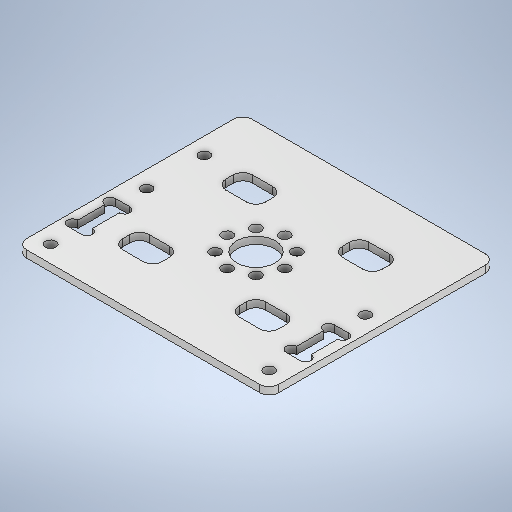
# Autodesk Inventor part: kosi_v3_1.5
Saved by Autodesk Inventor 2025.1 (Build 291241000, 241)
## iProperties
Created: 2024-09-01
Part Number: kosi_v3_1.5
Material: アルミニウム 2014-T4
Document SubType Name: Modeling
Designer: right
Density: 2.8 g/cm^3
Appearance: サテン
Mass: 8.90993 g
Surface Area: 49.4612 cm^2
Volume: 3.18212 cm^3
Author: right
Autodesk Inventor part; units mm, degrees
ref_plane "YZ Plane" through (0, 0, 0) normal (1, 0, 0) x (0, 1, 0)
ref_plane "XZ Plane" through (0, 0, 0) normal (0, 1, 0) x (-1, 0, 0)
ref_plane "XY Plane" through (0, 0, 0) normal (0, 0, 1) x (1, 0, 0)
sketch "スケッチ1" plane through (0, 0, 0) normal (0, 1, 0) x (-1, 0, 0)
  circle A0 centre (0, 0) radius 4
  circle A1 centre (0, 0) radius 8
  circle A2 centre (0, 0) radius 6 construction
  circle A3 centre (0, -6) radius 1.1
  circle A4 centre (4.2426, -4.2426) radius 1.1
  circle A5 centre (6, 0) radius 1.1
  circle A6 centre (4.2426, 4.2426) radius 1.1
  circle A7 centre (0, 6) radius 1.1
  circle A8 centre (-4.2426, 4.2426) radius 1.1
  circle A9 centre (-6, 0) radius 1.1
  circle A10 centre (-4.2426, -4.2426) radius 1.1
  line L0 (26.25, -23.5) -> (-26.25, -23.5)
  line L1 (-26.25, -23.5) -> (-26.25, 23.5)
  line L2 (-26.25, 23.5) -> (26.25, 23.5)
  line L3 (26.25, 23.5) -> (26.25, -23.5)
  line L4 (26.25, -23.5) -> (-26.25, 23.5) construction
  line L5 (-26.25, -23.5) -> (26.25, 23.5) construction
  line L6 (24.25, 5) -> (21.25, 5)
  line L7 (21.25, 5) -> (21.25, 15)
  line L8 (21.25, 15) -> (24.25, 15)
  line L9 (24.25, 15) -> (24.25, 5)
  circle A11 centre (24.25, 6.1) radius 1.1
  circle A12 centre (21.25, 6.1) radius 1.1
  line L10 (0, 0) -> (0, -23.5) construction
  circle A13 centre (24.25, 13.9) radius 1.1
  circle A14 centre (21.25, 13.9) radius 1.1
  line L11 (-24.25, 5) -> (-21.25, 5)
  line L12 (-21.25, 5) -> (-21.25, 15)
  line L13 (-21.25, 15) -> (-24.25, 15)
  line L14 (-24.25, 15) -> (-24.25, 5)
  circle A15 centre (-24.25, 6.1) radius 1.1
  circle A16 centre (-21.25, 6.1) radius 1.1
  circle A17 centre (-24.25, 13.9) radius 1.1
  circle A18 centre (-21.25, 13.9) radius 1.1
  circle A19 centre (22.75, 0) radius 1.1
  circle A20 centre (22.75, 20) radius 1.1
  circle A21 centre (-22.75, 0) radius 1.1
  circle A22 centre (-22.75, 20) radius 1.1
  circle A23 centre (22.75, 20) radius 3.5 construction
  point P0 (21.25, 10)
  point P1 (-21.25, 10)
  point P2 (22.75, 5)
  point P3 (-21.25, 12.8)
  point P4 (-21.25, 7.2)
  point P5 (-24.25, 7.2)
  point P6 (-24.25, 12.8)
  point P7 (-24.25, 15)
  point P8 (21.25, 12.8)
  point P9 (21.25, 15)
  point P10 (24.25, 15)
  point P11 (24.25, 12.8)
  point P12 (24.25, 7.2)
  point P13 (21.25, 7.2)
  point P14 (22.75, 15)
  dimension "d2" = 12
  dimension "d10" = 2.2
  dimension "d0" = 8
  dimension "d1" = 16
  dimension "d3" = 2.2
  dimension "d6" = 360
  dimension "d8" = 3
  dimension "d9" = 10
  dimension "d11" = 42.5
  dimension "d12" = 2.2
  dimension "d13" = 5
  dimension "d17" = 5
  dimension "d18" = 7
  constraints: 30 end point, 19 centre point, 11 symmetric about line, 7 midpoint, 6 point on line, 4 coincident, 4 parallel, 4 tangent, 4 vertical alignment, 2 equal radius, 2 horizontal, 2 perpendicular, 2 vertical, 1 horizontal alignment, 36 other
  measures "d0" diameter of A0
  measures "d1" diameter of A1
  measures "d3" diameter of A3
  measures "d8" distance of L6.start L6.end
  measures "d9" distance of L6.end L7.end
  measures "d11" distance between parallel lines of L12 L7
  measures "d12" diameter of A19
  measures "d13" distance from line of L6 A19.centre
  measures "d17" distance of point (22.75, 15) A20.centre
  measures "d18" diameter of A23
extrude "押し出し1" add sketch "スケッチ1" along normal blind 1.5 contours A1 | L0 L1 L2 L3
sketch "スケッチ2" plane through (0, 0, 0) normal (0, -1, 0) x (1, 0, 0)
  circle A0 centre (-22.75, -12) radius 1.1
  circle A1 centre (-22.75, 0) radius 1.1 projected
  point P0 (0, 0)
  dimension "d19" = 2.2
  dimension "d20" = 12
  constraints: 1 centre point, 1 vertical alignment
  measures "d19" diameter of A0
  measures "d20" distance of A0.centre A1.centre
extrude "押し出し2" cut sketch "スケッチ2" against normal through all contours A0
fillet "フィレット1" radius 2 4 edges at (-26.25, 0.75, -23.5) (26.25, 0.75, -23.5) (26.25, 0.75, 23.5) (-26.25, 0.75, 23.5)
sketch "スケッチ3" plane through (0, 1.5, 0) normal (0, 1, 0) x (1, 0, 0)
  arc A0 (-26.25, -21.5) -> (-24.25, -23.5) centre (-24.25, -21.5) ccw projected
  line L0 (-24.25, -23.5) -> (24.25, -23.5) projected
  arc A1 (24.25, -23.5) -> (26.25, -21.5) centre (24.25, -21.5) ccw projected
  line L1 (26.25, -21.5) -> (26.25, 21.5) projected
  arc A2 (26.25, 21.5) -> (24.25, 23.5) centre (24.25, 21.5) ccw projected
  line L2 (24.25, 23.5) -> (-24.25, 23.5) projected
  arc A3 (-24.25, 23.5) -> (-26.25, 21.5) centre (-24.25, 21.5) ccw projected
  line L3 (-26.25, 21.5) -> (-26.25, -21.5) projected
  circle A4 centre (-22.75, 12) radius 1.1 projected
  circle A5 centre (22.75, -20) radius 1.1 projected
  circle A6 centre (-22.75, -20) radius 1.1 projected
  circle A7 centre (-22.75, 0) radius 1.1 projected
  line L4 (21.25, -12.8) -> (21.25, -7.2) projected
  arc A8 (21.25, -5) -> (21.25, -7.2) centre (21.25, -6.1) ccw projected
  line L5 (21.25, -5) -> (24.25, -5) projected
  arc A9 (24.25, -7.2) -> (24.25, -5) centre (24.25, -6.1) ccw projected
  line L6 (24.25, -7.2) -> (24.25, -12.8) projected
  arc A10 (24.25, -15) -> (24.25, -12.8) centre (24.25, -13.9) ccw projected
  line L7 (24.25, -15) -> (21.25, -15) projected
  arc A11 (21.25, -12.8) -> (21.25, -15) centre (21.25, -13.9) ccw projected
  arc A12 (-21.25, -15) -> (-21.25, -12.8) centre (-21.25, -13.9) ccw projected
  line L8 (-21.25, -15) -> (-24.25, -15) projected
  arc A13 (-24.25, -12.8) -> (-24.25, -15) centre (-24.25, -13.9) ccw projected
  line L9 (-24.25, -12.8) -> (-24.25, -7.2) projected
  arc A14 (-24.25, -5) -> (-24.25, -7.2) centre (-24.25, -6.1) ccw projected
  line L10 (-24.25, -5) -> (-21.25, -5) projected
  arc A15 (-21.25, -7.2) -> (-21.25, -5) centre (-21.25, -6.1) ccw projected
  line L11 (-21.25, -7.2) -> (-21.25, -12.8) projected
  circle A16 centre (6, 0) radius 1.1 projected
  circle A17 centre (0, -6) radius 1.1 projected
  circle A18 centre (-6, 0) radius 1.1 projected
  circle A19 centre (0, 6) radius 1.1 projected
  circle A20 centre (22.75, 0) radius 1.1 projected
  circle A21 centre (4.2426, 4.2426) radius 1.1 projected
  circle A22 centre (4.2426, -4.2426) radius 1.1 projected
  circle A23 centre (-4.2426, -4.2426) radius 1.1 projected
  circle A24 centre (-4.2426, 4.2426) radius 1.1 projected
  circle A25 centre (0, 0) radius 4 projected
  circle A26 centre (0, 0) radius 8
  line L12 (-16.25, -13.5) -> (16.25, -13.5)
  line L13 (16.25, -13.5) -> (16.25, 13.5)
  line L14 (16.25, 13.5) -> (-16.25, 13.5)
  line L15 (-16.25, 13.5) -> (-16.25, -13.5)
  line L16 (-8, 0) -> (-8, -13.5)
  line L17 (8, 0) -> (8, -13.5)
  line L18 (-8, 0) -> (-8, 13.5)
  line L19 (8, 0) -> (8, 13.5)
  line L20 (0, -8) -> (-16.25, -8)
  line L21 (-16.25, 8) -> (0, 8)
  line L22 (0, 8) -> (16.25, 8)
  line L23 (0, -8) -> (16.25, -8)
  point P0 (-8, 8)
  point P1 (8, 8)
  point P2 (8, -8)
  point P3 (-8, -8)
  dimension "d24" = 16
  dimension "d25" = 10
  constraints: 24 end point, 8 point on line, 7 tangent, 5 perpendicular, 3 parallel, 3 point on circle, 1 centre point, 1 coincident, 3 other
  measures "d24" diameter of A26
  measures "d25" distance between parallel lines of L3 L15
extrude "押し出し3" cut sketch "スケッチ3" against normal through all contours L23 L13 L12 L17 | L19 L14 L13 L22 | L21 L15 L14 L18 | L16 L12 L15 L20
fillet "フィレット2" radius 2 16 edges at (-16.25, 0.75, 8) (-16.25, 0.75, 13.5) (-8, 0.75, 13.5) (-8, 0.75, 8) (8, 0.75, 13.5) (16.25, 0.75, 13.5) (16.25, 0.75, 8) (8, 0.75, 8) (16.25, 0.75, -8) (16.25, 0.75, -13.5) (8, 0.75, -13.5) (8, 0.75, -8) (-8, 0.75, -8) (-16.25, 0.75, -13.5) (-16.25, 0.75, -8) (-8, 0.75, -13.5)
equation "\"d17\" = d13"
